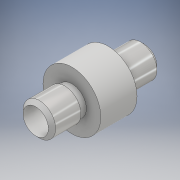
# Autodesk Inventor part: reverse gear cylinder piping connector 2
Saved by Autodesk Inventor 2017 (Build 210142000, 142)
## iProperties
Created: 2018-11-06
Part Number: reverse gear cylinder piping connector 2
Material: Generic
Document SubType Name: Modeling
Designer: User
Density: 1 g/cm^3
Appearance: Default
Author: User
Autodesk Inventor part; units mm, degrees
ref_plane "YZ Plane" through (0, 0, 0) normal (1, 0, 0) x (0, 1, 0)
ref_plane "XY Plane" through (0, 0, 0) normal (0, 0, 1) x (1, 0, 0)
sketch "Sketch1" plane through (0, 0, 0) normal (0, 1, 0) x (-1, 0, 0)
  circle A0 centre (0, 0) radius 1.75
  circle A1 centre (0, 0) radius 2
  dimension "d0" = 3.5
  dimension "d1" = 4
  constraints: 2 centre point, 2 coincident
  measures "d0" diameter of A0
  measures "d1" diameter of A1
extrude "Extrusion1" add sketch "Sketch1" along normal blind 15
sketch "Sketch2" plane through (0, 0, 0) normal (0, -1, 0) x (1, 0, 0)
  circle A0 centre (0, 0) radius 2.25
  circle A1 centre (0, 0) radius 2
  dimension "d4" = 4.5
  constraints: 2 centre point, 2 coincident
  measures "d4" diameter of A0
extrude "Extrusion2" add sketch "Sketch2" against normal blind 4
sketch "Sketch3" plane through (0, 15, 0) normal (0, 1, 0) x (1, 0, 0)
  circle A0 centre (0, 0) radius 2
  circle A1 centre (0, 0) radius 2.25
  circle A2 centre (0, 0) radius 2.25
  dimension "d9" = 4.5
  dimension "d10" = 4.5
  dimension "d11" = 4
  dimension "d12" = 0
  constraints: 3 centre point, 2 coincident, 1 concentric
  measures "d9" diameter of A2
  measures "d10" diameter of A1
  measures "d11" diameter of A0
  measures "d12" distance of point (0, 0) A2.centre
extrude "Extrusion3" add sketch "Sketch3" against normal blind 4
ref_plane "Work Plane4" through (0, 7.5, 0) normal (0, 1, 0) x (-1, 0, 0)
ref_plane "Work Plane3" through (0, -4, 0) normal (0, 1, 0) x (-1, 0, 0)
sketch "Sketch4" plane through (0, 7.5, 0) normal (0, 1, 0) x (-1, 0, 0)
  circle A0 centre (0, 0) radius 2
  circle A1 centre (0, 0) radius 4
  dimension "d16" = 4
  dimension "d17" = 8
  constraints: 2 centre point, 2 coincident
  measures "d16" diameter of A0
  measures "d17" diameter of A1
chamfer "Chamfer3" distance 0.5 angle 45 1 edges at (-2.25, 0, 0)
chamfer "Chamfer4" distance 0.5 angle 45 1 edges at (-2.25, 15, 0)
extrude "Extrusion5" add sketch "Sketch4" along normal mid plane 5
body "Solid1"
